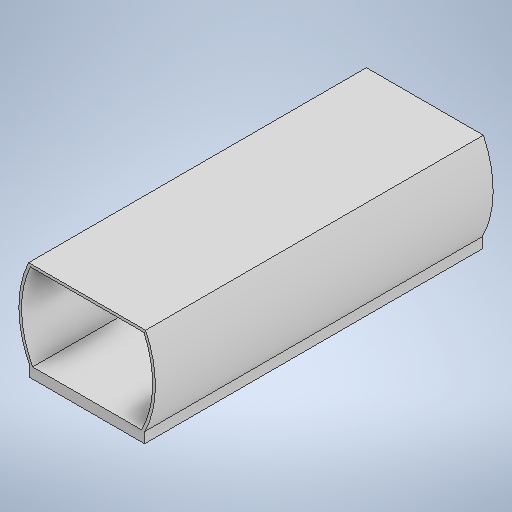
# Autodesk Inventor part: PCB Battery Tray
Saved by Autodesk Inventor 2025 (Build 290162000, 162)
## iProperties
Created: 2024-07-12
Part Number: PCB Battery Tray
Material: Generic
Document SubType Name: Modeling
Designer: track
Density: 1 g/cm^3
Appearance: Default
Author: track
## iProperties of the stored document PCB Battery Tray_3DPrint.ipt
Created: 2024-07-12
Part Number: PCB Battery Tray_3DPrint
Material: Generic
Document SubType Name: Modeling
Designer: track
Density: 1 g/cm^3
Appearance: Default
Author: track
Autodesk Inventor part; units mm, degrees
ref_plane "YZ Plane" through (0, 0, 0) normal (1, 0, 0) x (0, 1, 0)
ref_plane "XZ Plane" through (0, 0, 0) normal (0, 1, 0) x (-1, 0, 0)
ref_plane "XY Plane" through (0, 0, 0) normal (0, 0, 1) x (1, 0, 0)
sketch "Sketch1" plane through (0, 0, 0) normal (0, 0, 1) x (1, 0, 0)
  line L0 (0, 0) -> (0, 2.54)
  line L1 (0, 2.54) -> (35.6964, 2.54)
  line L2 (35.6964, 2.54) -> (35.6964, 0)
  line L3 (-0.889, 0) -> (-0.889, 3.429)
  line L4 (-0.889, 3.429) -> (36.5854, 3.429)
  line L5 (36.5854, 3.429) -> (36.5854, 0)
  line L6 (-0.889, 0) -> (0, 0)
  line L7 (35.6964, 0) -> (36.5854, 0)
  line L8 (36.8982, 32.179) -> (-1.2018, 32.179)
  arc A0 (36.5854, 3.429) -> (36.8982, 32.179) centre (7.3744, 18.1235) ccw
  line L9 (17.8482, 3.429) -> (17.8482, 32.179) construction
  arc A1 (-1.2018, 32.179) -> (-0.889, 3.429) centre (28.322, 18.1235) ccw
  line L10 (40.0732, 18.1235) -> (-4.3768, 18.1235)
  arc A2 (35.5867, 3.429) -> (36.3314, 31.29) centre (7.3744, 18.1235) ccw
  line L11 (36.3314, 31.29) -> (-0.635, 31.29)
  arc A3 (-0.635, 31.29) -> (0.1097, 3.429) centre (28.322, 18.1235) ccw
  dimension "d0" = 35.6964
  dimension "d1" = 2.54
  dimension "d2" = 2.54
  dimension "d3" = 0.889
  dimension "d11" = 28.75
  dimension "d14" = 38.1
  dimension "d15" = 0
  dimension "d16" = 44.45
  dimension "d17" = 0.889
  constraints: 24 end point, 10 point on circle, 4 centre point, 4 perpendicular, 3 horizontal, 2 midpoint, 2 point on line, 1 collinear, 1 vertical, 5 other
  measures "d0" distance of L0.end L1.end
  measures "d1" distance of L1.end L2.end
  measures "d2" distance of L0.start L0.end
  measures "d3" distance between parallel lines of L3 L0
  measures "d11" distance between parallel lines of L4 L8
  measures "d14" distance of L8.start L8.end
  measures "d15" distance from line of A0.centre L10
  measures "d16" distance of L10.start L10.end
  measures "d17" radial gap between concentric circles of A0 A2
extrude "Extrusion1" add sketch "Sketch1" against normal blind 110 contours L6 L3 L4 L5 L7 L2 L1 L0 | A1 L10 A3 L4 | A1 L8 A0 L10 A2 L11 A3 | A2 L10 A0 L4
sketch "Sketch2" plane through (0, 0, 0) normal (0, 0, 1) x (1, 0, 0)
  line L0 (-0.889, 3.429) -> (36.5854, 3.429)
  line L1 (36.5854, 3.429) -> (36.5854, 0)
  line L2 (36.5854, 0) -> (-0.889, 0)
  line L3 (-0.889, 0) -> (-0.889, 3.429)
  line L4 (36.5854, 0) -> (36.5854, 3.429) projected
  line L5 (35.6964, 0) -> (36.5854, 0) projected
  line L6 (35.5867, 3.429) -> (0.1097, 3.429) projected
  line L7 (-0.889, 3.429) -> (-0.889, 0) projected
  constraints: 8 end point, 4 collinear, 2 parallel, 1 horizontal, 1 perpendicular
extrude "Extrusion2" add sketch "Sketch2" against normal blind 1
body "Solid1"
